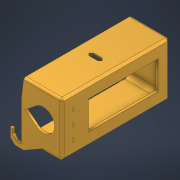
# Autodesk Inventor part: Mount Case
Saved by Autodesk Inventor 2022 (Build 260153000, 153)
## iProperties
Created: 2021-08-06
Part Number: Mount Case
Material: Generic
Document SubType Name: Modeling
Designer: sidsa
Density: 1 g/cm^3
Appearance: Brass - Satin
Author: sidsa
## iProperties of the stored document Mount Case_3DPrint.ipt
Created: 2021-08-06
Part Number: Mount Case_3DPrint
Material: Generic
Document SubType Name: Modeling
Designer: sidsa
Density: 1 g/cm^3
Appearance: Default
Author: sidsa
Autodesk Inventor part; units mm, degrees
ref_plane "YZ Plane" through (0, 0, 0) normal (1, 0, 0) x (0, 1, 0)
ref_plane "XZ Plane" through (0, 0, 0) normal (0, 1, 0) x (-1, 0, 0)
sketch "Sketch1" plane through (0, 0, 0) normal (1, 0, 0) x (0, 1, 0)
  line L0 (0, 0) -> (76.2, 0)
  line L1 (76.2, 0) -> (76.2, -152.4)
  line L2 (76.2, -152.4) -> (0, -152.4)
  line L3 (0, -152.4) -> (0, 0)
  line L4 (38.1, -152.4) -> (38.1, 0)
  line L5 (18.0975, -135.89) -> (18.0975, -38.1)
  line L6 (18.0975, -38.1) -> (58.1025, -38.1)
  line L7 (58.1025, -38.1) -> (58.1025, -135.89)
  line L8 (58.1025, -135.89) -> (18.0975, -135.89)
  line L9 (18.0975, -135.89) -> (58.1025, -38.1) construction
  line L10 (18.0975, -38.1) -> (58.1025, -135.89) construction
  point P0 (38.1, -86.995)
  dimension "d0" = 152.4
  dimension "d1" = 76.2
  dimension "d4" = 97.79
  dimension "d5" = 40.005
  dimension "d6" = 38.1
  constraints: 22 end point, 4 midpoint, 4 parallel, 2 perpendicular, 1 horizontal, 1 point on line
  measures "d0" distance of L0.end L1.end
  measures "d1" distance of L1.end L2.end
  measures "d4" distance of L5.start L5.end
  measures "d5" distance of L5.end L6.end
  measures "d6" distance between parallel lines of L0 L6
extrude "Extrusion1" add sketch "Sketch1" against normal blind 3.175 contours L0 L4 L6 L5 L8 L2 L3 | L0 L1 L2 L4 L8 L7 L6
sketch "Sketch2" plane through (-3.175, 0, 0) normal (-1, 0, 0) x (0, 0, 1)
  line L0 (-152.4, 0) -> (0, 0) projected
  line L1 (0, 0) -> (0, 76.2) projected
  line L2 (0, 76.2) -> (-152.4, 76.2) projected
  line L3 (-152.4, 76.2) -> (-152.4, 0) projected
  line L4 (-38.1, 58.1025) -> (-38.1, 18.0975) projected
  line L5 (-38.1, 18.0975) -> (-135.89, 18.0975) projected
  line L6 (-135.89, 18.0975) -> (-135.89, 58.1025) projected
  line L7 (-135.89, 58.1025) -> (-38.1, 58.1025) projected
  line L8 (-3.175, 73.025) -> (-3.175, 3.175)
  line L9 (-3.175, 3.175) -> (-149.225, 3.175)
  line L10 (-149.225, 3.175) -> (-149.225, 73.025)
  line L11 (-149.225, 73.025) -> (-3.175, 73.025)
  dimension "d9" = 3.175
  constraints: 8 end point, 3 other
  measures "d9" distance between parallel lines of L1 L8
extrude "Extrusion2" add sketch "Sketch2" along normal blind 50.8 contours L3 L2 L1 L0
sketch "Sketch3" plane through (0, 0, -152.4) normal (0, 0, -1) x (-1, 0, 0)
  line L0 (0, 0) -> (53.975, 0) projected
  line L1 (53.975, 0) -> (53.975, -12.7)
  line L2 (53.975, -12.7) -> (66.675, -12.7)
  line L3 (66.675, -12.7) -> (73.025, -6.35)
  line L4 (73.025, -6.35) -> (73.025, 6.35)
  line L5 (73.025, 6.35) -> (69.85, 6.35)
  line L6 (69.85, 6.35) -> (69.85, -0.5447)
  line L7 (69.85, -0.5447) -> (64.0447, -6.35)
  line L8 (64.0447, -6.35) -> (57.15, -6.35)
  line L9 (57.15, -6.35) -> (57.15, 0)
  line L10 (57.15, 0) -> (57.15, 50.8)
  line L11 (0, 76.2) -> (53.975, 76.2) projected
  line L12 (57.15, 50.8) -> (53.975, 76.2)
  line L13 (53.975, -12.7) -> (31.978, 0)
  line L14 (0, 0) -> (0, 76.2) projected
  line L15 (0, 0) -> (53.975, 0) projected
  line L16 (53.975, 76.2) -> (53.975, 0) projected
  line L17 (0, 76.2) -> (53.975, 76.2) projected
  dimension "d12" = 12.7
  dimension "d15" = 12.7
  dimension "d16" = 3.175
  dimension "d17" = 50.8
  dimension "d18" = 3.175
  dimension "d19" = 6.35
  dimension "d20" = 6.35
  dimension "d21" = 12.7
  dimension "d22" = 6.35
  dimension "d23" = 135
  dimension "d24" = 25.4
  constraints: 24 end point, 4 perpendicular, 2 parallel, 2 point on line, 2 vertical
  measures "d12" distance of L0.end L1.end
  measures "d15" distance of L3.end L4.end
  measures "d16" distance of L4.end L5.end
  measures "d17" distance of L9.end L10.end
  measures "d18" distance between parallel lines of L1 L9
  measures "d19" distance between parallel lines of L2 L8
  measures "d20" distance between parallel lines of L3 L7
  measures "d21" distance of L1.end L2.end
  measures "d22" horizontal distance of L2.end L3.end
  measures "d23" angle of L2 L3
  measures "d24" distance of L1.end L13.end
extrude "Extrusion3" add sketch "Sketch3" against normal blind 3.175 contours L0 L1 L13 | L16 L12 L10 L9 L8 L7 L6 L5 L4 L3 L2 L1
ref_plane "Work Plane1" through (0, 0, -76.2) normal (0, 0, -1) x (-1, 0, 0)
mirror "Mirror1" about plane through (0, 0, -76.2) normal (0, 0, -1) of "Extrusion3"
sketch "Sketch4" plane through (0, 0, -152.4) normal (0, 0, -1) x (-1, 0, 0)
  line L0 (0, 0) -> (0, 76.2) projected
  line L1 (0, 0) -> (31.978, 0) projected
  line L2 (31.978, 0) -> (53.975, -12.7) projected
  line L3 (53.975, -12.7) -> (66.675, -12.7) projected
  line L4 (66.675, -12.7) -> (73.025, -6.35) projected
  line L5 (73.025, -6.35) -> (73.025, 6.35) projected
  line L6 (73.025, 6.35) -> (69.85, 6.35) projected
  line L7 (69.85, 6.35) -> (69.85, -0.5447) projected
  line L8 (69.85, -0.5447) -> (64.0447, -6.35) projected
  line L9 (64.0447, -6.35) -> (57.15, -6.35) projected
  line L10 (57.15, -6.35) -> (57.15, 50.8) projected
  line L11 (57.15, 50.8) -> (53.975, 76.2) projected
  line L12 (0, 76.2) -> (53.975, 76.2) projected
  line L13 (7.62, 68.58) -> (7.62, 7.62)
  line L14 (7.62, 7.62) -> (34.0197, 7.62)
  line L15 (34.0197, 7.62) -> (49.53, -1.3349)
  line L16 (49.53, -1.3349) -> (49.53, 50.3256)
  line L17 (49.53, 50.3256) -> (47.2482, 68.58)
  line L18 (47.2482, 68.58) -> (7.62, 68.58)
  line L19 (49.53, 49.8475) -> (7.62, 49.8475)
  line L20 (10.4775, 49.8475) -> (10.4775, 68.58)
  point P0 (0, 0)
  dimension "d27" = 7.62
  constraints: 16 end point, 4 point on line, 2 perpendicular, 5 other
  measures "d27" distance between parallel lines of L0 L13
extrude "Extrusion4" cut sketch "Sketch4" against normal blind 3.175 contours L18 L20 L19 L13
fillet "Fillet1" radius 3.175 4 edges at (-15.989, 0, -152.4) (-15.989, 0, 0) (-26.9875, 76.2, -152.4) (-26.9875, 76.2, 0)
chamfer "Chamfer1" distance 0.3969 angle 45 4 edges at (0, 38.1, -38.1) (0, 18.0975, -86.995) (0, 58.1025, -86.995) (0, 38.1, -135.89)
chamfer "Chamfer2" distance 3.175 angle 45 8 edges at (0, 0, -76.2) (0, 0.9299, -151.4701) (0, 38.1, -152.4) (0, 75.2701, -151.4701) (0, 76.2, -76.2) (0, 75.2701, -0.9299) (0, 38.1, 0) (0, 0.9299, -0.9299)
pattern_linear "Rectangular Pattern1" count 5 spacing 9.525 along (-1, 0, 0) of "Extrusion4"
fillet "Fillet2" radius 6.35 2 edges at (-42.9765, 0, -3.175) (-42.9765, 0, -149.225)
fillet "Fillet3" radius 6.35 4 edges at (-53.975, -3.175, -3.175) (-53.975, 1.5875, -3.175) (-53.975, -3.175, -149.225) (-53.975, 1.5875, -149.225)
sketch "Sketch6" plane through (-66.675, -12.7, 0) normal (0, 0, 1) x (1, 0, 0)
  line L0 (63.5, 85.725) -> (63.5, 15.875) projected
  line L1 (12.3031, 85.725) -> (63.5, 85.725) projected
  line L2 (9.525, 63.5) -> (12.3031, 85.725) projected
  line L3 (9.525, 6.35) -> (9.525, 63.5) projected
  line L4 (2.6303, 6.35) -> (9.525, 6.35) projected
  line L5 (-3.175, 12.1553) -> (2.6303, 6.35) projected
  line L6 (-3.175, 19.05) -> (-3.175, 12.1553) projected
  line L7 (-6.35, 19.05) -> (-3.175, 19.05) projected
  line L8 (-6.35, 6.35) -> (-6.35, 19.05) projected
  line L9 (0, 0) -> (-6.35, 6.35) projected
  line L10 (12.7, 0) -> (0, 0) projected
  line L11 (40.1963, 15.875) -> (12.7, 0) projected
  line L12 (63.5, 15.875) -> (40.1963, 15.875) projected
  line L13 (40.1963, 15.875) -> (40.1963, 85.725) construction
  line L14 (63.5, 85.725) -> (12.7, 85.725) construction
  circle A0 centre (40.1963, 50.8) radius 16.002
  line L15 (40.1963, 50.8) -> (14.7963, 50.8) construction
  line L16 (14.7963, 50.8) -> (30.115, 38.3729)
  line L17 (14.7963, 50.8) -> (30.115, 63.2271)
  point P0 (66.675, 12.7)
  dimension "d47" = 32.004
  dimension "d48" = 25.4
  constraints: 8 end point, 2 point on circle, 2 tangent, 1 centre point, 1 horizontal, 1 midpoint, 1 perpendicular, 1 point on line
  measures "d47" diameter of A0
  measures "d48" distance of L15.start L15.end
extrude "Extrusion6" cut sketch "Sketch6" against normal blind 25.4 contours A0 | A0 L16 L17
sketch "Sketch7" plane through (-53.975, 76.2, -3.175) normal (0, 1, 0) x (1, 0, 0)
  line L0 (50.8, 146.05) -> (50.8, 0) projected
  line L1 (0, 146.05) -> (50.8, 146.05) projected
  line L2 (0, 0) -> (0, 146.05) projected
  line L3 (50.8, 0) -> (0, 0) projected
  line L4 (50.8, 132.715) -> (50.8, 34.925) construction
  line L5 (50.8, 73.025) -> (0, 73.025) construction
  line L6 (0, 139.7) -> (0, 6.35) construction
  line L7 (34.925, 76.2) -> (15.875, 76.2)
  line L8 (15.875, 76.2) -> (15.875, 69.85)
  line L9 (15.875, 69.85) -> (34.925, 69.85)
  line L10 (34.925, 69.85) -> (34.925, 76.2)
  line L11 (34.925, 76.2) -> (15.875, 69.85) construction
  line L12 (15.875, 76.2) -> (34.925, 69.85) construction
  point P0 (53.975, -3.175)
  point P1 (25.4, 73.025)
  dimension "d51" = 19.05
  dimension "d52" = 6.35
  constraints: 14 end point, 4 midpoint, 2 parallel, 1 perpendicular, 1 point on line
  measures "d51" distance of L7.start L7.end
  measures "d52" distance of L8.end L7.end
extrude "Extrusion7" cut sketch "Sketch7" against normal blind 25.4 contours L10 L9 L8 L7
chamfer "Chamfer3" distance 3.175 angle 45 4 edges at (-19.05, 74.6125, -79.375) (-19.05, 74.6125, -73.025) (-38.1, 74.6125, -73.025) (-38.1, 74.6125, -79.375)
sketch "Sketch8" plane through (0, 0, 0) normal (1, 0, 0) x (0, 0, -1)
  circle A0 centre (15.875, 35.56) radius 0.635
  circle A1 centre (15.875, 39.37) radius 0.635
  line L0 (15.875, 15.875) -> (15.875, 34.925) construction
  line L1 (37.7031, 58.4994) -> (37.7031, 17.7006) construction
  line L2 (37.7031, 37.465) -> (3.175, 37.465) construction
  line L3 (3.175, 3.175) -> (3.175, 73.025) construction
  circle A2 centre (15.875, 54.61) radius 0.635
  circle A3 centre (15.875, 58.42) radius 0.635
  circle A4 centre (15.875, 16.51) radius 0.635
  circle A5 centre (15.875, 20.32) radius 0.635
  circle A6 centre (15.875, 35.56) radius 0.635
  circle A7 centre (15.875, 39.37) radius 0.635
  point P0 (0, 0)
  point P1 (15.875, 37.465)
  point P2 (15.875, 56.515)
  point P3 (15.875, 53.975)
  point P4 (15.875, 18.415)
  point P5 (15.875, 37.465)
  dimension "d61" = 1.905
  dimension "d62" = 1.905
  dimension "d63" = 0
  dimension "d64" = 12.7
  dimension "d67" = 19.05
  dimension "d70" = 19.05
  constraints: 8 centre point, 4 end point, 3 vertical, 1 horizontal, 1 point on line, 18 other
  measures "d61" distance of point (15.875, 37.465) A0.centre
  measures "d62" distance of point (15.875, 37.465) A1.centre
  measures "d63" distance from line of point (15.875, 37.465) L2
  measures "d64" distance from line of L3 A1.centre
  measures "d67" distance of point (15.875, 37.465) point (15.875, 56.515)
  measures "d70" distance of point (15.875, 37.465) point (15.875, 18.415)
extrude "Extrusion8" cut sketch "Sketch8" against normal blind 25.4
fillet "Fillet4" radius 6.35 4 edges at (-30.1625, 3.175, -3.175) (-28.575, 73.025, -3.175) (-30.1625, 3.175, -149.225) (-28.575, 73.025, -149.225)
equation "\"d49\" = d48"
equation "\"d53\" = d48"
equation "\"d73\" = d48"
body "Solid1"
